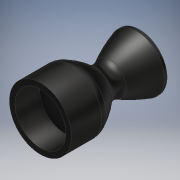
# Autodesk Inventor part: nozzle-cfd
Saved by Autodesk Inventor 2017 (Build 210142000, 142)
## iProperties
Created: 2020-06-17
Part Number: nozzle-cfd
Material: ABS Plastic
Document SubType Name: Modeling
Designer: HAYNIE R&D
Density: 1.06 g/cm^3
Appearance: Smooth - White
Author: HAYNIE R&D
Autodesk Inventor part; units mm, degrees
ref_plane "YZ Plane" through (0, 0, 0) normal (1, 0, 0) x (0, 1, 0)
ref_plane "XZ Plane" through (0, 0, 0) normal (0, 1, 0) x (-1, 0, 0)
ref_plane "XY Plane" through (0, 0, 0) normal (0, 0, 1) x (1, 0, 0)
sketch "Sketch1" plane through (0, 0, 0) normal (1, 0, 0) x (0, 1, 0)
  line L0 (9.25, 0.0185) -> (11.25, 0.0185)
  line L1 (11.25, 0.0185) -> (11.25, -9.9815)
  line L2 (11.25, -9.9815) -> (11.25, -12)
  arc A0 (1.9984, -22.0011) -> (7.875, -14) centre (-8.063, -8.4526) ccw
  arc A1 (7.9841, -34.947) -> (1.9984, -22.0011) centre (-30.628, -44.9433) ccw
  arc A2 (4, -22) -> (11.25, -12) centre (-13.1002, -1.9743) ccw
  arc A3 (9.9841, -34.947) -> (4, -22) centre (-38.5, -49.5) ccw
  line L3 (7.875, -9.9815) -> (7.875, -14)
  line L4 (0, 0) -> (0, -36)
  line L5 (7.9841, -34.947) -> (0, -34.947)
  line L6 (0, -34.947) -> (0, -35.947)
  line L7 (9.9841, -34.947) -> (9.9841, -35.947)
  line L8 (9.9841, -35.947) -> (0, -35.947)
  line L9 (7.875, -9.9815) -> (0, -9.9815)
  line L10 (0, -9.9815) -> (0, -8.9815)
  line L11 (0, -8.9815) -> (9.25, -8.9815)
  line L12 (9.25, -8.9815) -> (9.25, 0.0185)
  dimension "d26" = 9.25
  dimension "d28" = 2
  dimension "d37" = 34.9656
  dimension "d57" = 36
  dimension "d59" = 1
  dimension "d60" = 1
  dimension "d61" = 90
  constraints: 26 end point, 8 point on circle, 4 centre point, 4 perpendicular, 4 vertical, 3 point on line, 1 horizontal
  measures "d26" distance of L4.start L0.start
  measures "d28" distance of L0.start L0.end
  measures "d37" vertical distance of L7.start L0.end
  measures "d57" distance of L4.start L4.end
  measures "d59" distance of L5.end L6.end
  measures "d60" distance of L9.end L10.end
  measures "d61" angle of L10 L11
revolve "Revolution1" add sketch "Sketch1" angle 360 about axis through (0, 0, 0) along (0, 0, -1) contours L0 L1 L2 A2 A3 L7 L8 L4 L5 A1 A0 L3 L9 L11 L12
move or copy body "Move Body1" bodies to move or copy 1 copy no rotation origin (0, 0, 0) rotation axis (1, 0, 0) rotation angle 90
fillet "Fillet6" radius 2 1 edges at (0, 22.0011, -1.9984)
fillet "Fillet7" radius 5 1 edges at (0, 14, -7.875)
fillet "Fillet8" radius 5 1 edges at (0, 12, -11.25)
fillet "Fillet9" radius 5 1 edges at (0, 22, -4)
body "Solid1"
